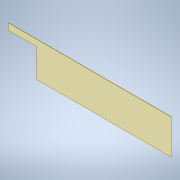
# Autodesk Inventor part: cover back
Saved by Autodesk Inventor 2021 (Build 250183000, 183)
## iProperties
Created: 2024-06-13
Part Number: cover back
Material: Nylon 6/6
Document SubType Name: Modeling
Designer: ASUS
Density: 1.13 g/cm^3
Appearance: Nylon 6
Author: ASUS
Autodesk Inventor part; units mm, degrees
ref_plane "YZ Plane" through (0, 0, 0) normal (1, 0, 0) x (0, 1, 0)
ref_plane "XZ Plane" through (0, 0, 0) normal (0, 1, 0) x (-1, 0, 0)
ref_plane "XY Plane" through (0, 0, 0) normal (0, 0, 1) x (1, 0, 0)
sketch "Sketch1" plane through (0, 0, 0) normal (0, 0, 1) x (1, 0, 0)
  line L0 (0, 0) -> (2000, 0)
  line L1 (2000, 0) -> (2000, 427)
  line L2 (2000, 427) -> (0, 427)
  line L3 (0, 427) -> (0, 0)
  dimension "d0" = 2000
  dimension "d1" = 427
  constraints: 8 end point, 2 parallel, 1 horizontal, 1 perpendicular
  measures "d0" distance between parallel lines of L1 L3
  measures "d1" distance between parallel lines of L0 L2
extrude "Extrusion1" add sketch "Sketch1" along normal blind 3
sketch "Sketch2" plane through (0, 0, 3) normal (0, 0, 1) x (1, 0, 0)
  line L0 (0, 427) -> (0, 0) projected
  line L1 (0, 0) -> (350, 0)
  line L2 (350, 0) -> (350, 350)
  line L3 (350, 350) -> (0, 350)
  line L4 (0, 350) -> (0, 0)
  point P0 (0, 350)
  dimension "d4" = 350
  dimension "d5" = 350
  constraints: 8 end point, 2 parallel, 1 horizontal, 1 perpendicular
  measures "d4" distance between parallel lines of L1 L3
  measures "d5" distance between parallel lines of L2 L0
extrude "Extrusion2" cut sketch "Sketch2" against normal blind 10
body "Solid1"
